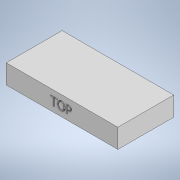
# Autodesk Inventor part: cable_jig_3.5_shim
Saved by Autodesk Inventor 2022 (Build 260153000, 153)
## iProperties
Created: 2022-03-09
Part Number: cable_jig_3.5_shim
Material: Generic
Document SubType Name: Modeling
Designer: kylem
Density: 1 g/cm^3
Appearance: Default
Author: kylem
Autodesk Inventor part; units mm, degrees
ref_plane "YZ Plane" through (0, 0, 0) normal (1, 0, 0) x (0, 1, 0)
ref_plane "XZ Plane" through (0, 0, 0) normal (0, 1, 0) x (-1, 0, 0)
ref_plane "XY Plane" through (0, 0, 0) normal (0, 0, 1) x (1, 0, 0)
sketch "Sketch1" plane through (0, 0, 0) normal (0, 1, 0) x (-1, 0, 0)
  line L0 (0, 0) -> (20, 0)
  line L1 (20, 0) -> (20, -10)
  line L2 (20, -10) -> (0, -10)
  line L3 (0, -10) -> (0, 0)
  dimension "d0" = 20
  dimension "d1" = 10
  constraints: 8 end point, 2 parallel, 1 horizontal, 1 perpendicular
  measures "d0" distance of L1.end L2.end
  measures "d1" distance of L0.end L1.end
extrude "Extrusion1" add sketch "Sketch1" along normal blind 3.45
sketch "Sketch2" plane through (-20, 0, 0) normal (0, 0, 1) x (1, 0, 0)
  line L0 (7.9399, 2.49) -> (16.3941, 2.49) construction
  line L1 (16.3941, 2.49) -> (16.3941, 0.9734) construction
  line L2 (16.3941, 0.9734) -> (7.9399, 0.9734) construction
  line L3 (7.9399, 0.9734) -> (7.9399, 2.49) construction
  line L4 (8.4419, 0.9584) -> (8.4419, 2.2809)
  line L5 (8.4419, 2.2809) -> (7.9386, 2.2809)
  line L6 (7.9386, 2.2809) -> (7.9386, 2.4584)
  line L7 (7.9386, 2.4584) -> (9.1445, 2.4584)
  line L8 (9.1445, 2.4584) -> (9.1445, 2.2809)
  line L9 (9.1445, 2.2809) -> (8.6412, 2.2809)
  line L10 (8.6412, 2.2809) -> (8.6412, 0.9584)
  line L11 (8.6412, 0.9584) -> (8.4419, 0.9584)
  spline S0 degree 2 poles (10.3576, 2.287) (10.4427, 2.1873) (10.5375, 1.8956) (10.5375, 1.7084) knots 0 0 0 1 2 2 2
  spline S1 degree 2 poles (10.5375, 1.7084) (10.5375, 1.526) (10.4451, 1.2307) (10.3576, 1.131) knots 0 0 0 1 2 2 2
  spline S2 degree 2 poles (10.3576, 1.131) (10.2652, 1.0264) (10.0209, 0.9268) (9.8738, 0.9268) knots 0 0 0 1 2 2 2
  spline S3 degree 2 poles (9.8738, 0.9268) (9.7219, 0.9268) (9.4788, 1.0301) (9.39, 1.131) knots 0 0 0 1 2 2 2
  spline S4 degree 2 poles (9.39, 1.131) (9.3037, 1.2307) (9.2113, 1.5236) (9.2113, 1.7084) knots 0 0 0 1 2 2 2
  spline S5 degree 2 poles (9.2113, 1.7084) (9.2113, 1.8968) (9.3049, 2.1837) (9.3912, 2.287) knots 0 0 0 1 2 2 2
  spline S6 degree 2 poles (9.3912, 2.287) (9.4788, 2.3867) (9.7231, 2.49) (9.8738, 2.49) knots 0 0 0 1 2 2 2
  spline S7 degree 2 poles (9.8738, 2.49) (10.027, 2.49) (10.2725, 2.383) (10.3576, 2.287) knots 0 0 0 1 2 2 2
  spline S8 degree 2 poles (10.3296, 1.7084) (10.3296, 1.8567) (10.2652, 2.0864) (10.2069, 2.1618) knots 0 0 0 1 2 2 2
  spline S9 degree 2 poles (10.2069, 2.1618) (10.1473, 2.2396) (9.9796, 2.3174) (9.875, 2.3174) knots 0 0 0 1 2 2 2
  spline S10 degree 2 poles (9.875, 2.3174) (9.7668, 2.3174) (9.604, 2.242) (9.542, 2.1618) knots 0 0 0 1 2 2 2
  spline S11 degree 2 poles (9.542, 2.1618) (9.4824, 2.0852) (9.4192, 1.8542) (9.4192, 1.7084) knots 0 0 0 1 2 2 2
  spline S12 degree 2 poles (9.4192, 1.7084) (9.4192, 1.413) (9.6672, 1.0994) (9.875, 1.0994) knots 0 0 0 1 2 2 2
  spline S13 degree 2 poles (9.875, 1.0994) (10.0829, 1.0994) (10.3296, 1.413) (10.3296, 1.7084) knots 0 0 0 1 2 2 2
  spline S14 degree 2 poles (11.7044, 2.0062) (11.7044, 1.9089) (11.6352, 1.7339) (11.5732, 1.6731) knots 0 0 0 1 2 2 2
  spline S15 degree 2 poles (11.5732, 1.6731) (11.4954, 1.5965) (11.2851, 1.5175) (11.1246, 1.5175) knots 0 0 0 1 2 2 2
  line L12 (11.1246, 1.5175) -> (10.9557, 1.5175)
  line L13 (10.9557, 1.5175) -> (10.9557, 0.9584)
  line L14 (10.9557, 0.9584) -> (10.7563, 0.9584)
  line L15 (10.7563, 0.9584) -> (10.7563, 2.4584)
  line L16 (10.7563, 2.4584) -> (11.1331, 2.4584)
  spline S16 degree 2 poles (11.1331, 2.4584) (11.2668, 2.4584) (11.454, 2.4146) (11.5258, 2.3648) knots 0 0 0 1 2 2 2
  spline S17 degree 2 poles (11.5258, 2.3648) (11.6096, 2.3076) (11.7044, 2.1314) (11.7044, 2.0062) knots 0 0 0 1 2 2 2
  spline S18 degree 2 poles (11.4966, 2.0001) (11.4966, 2.0779) (11.4431, 2.1922) (11.3884, 2.2286) knots 0 0 0 1 2 2 2
  spline S19 degree 2 poles (11.3884, 2.2286) (11.341, 2.2602) (11.2146, 2.2858) (11.121, 2.2858) knots 0 0 0 1 2 2 2
  line L17 (11.121, 2.2858) -> (10.9557, 2.2858)
  line L18 (10.9557, 2.2858) -> (10.9557, 1.6877)
  line L19 (10.9557, 1.6877) -> (11.0918, 1.6877)
  spline S20 degree 2 poles (11.0918, 1.6877) (11.2134, 1.6877) (11.3629, 1.7266) (11.4115, 1.7777) knots 0 0 0 1 2 2 2
  spline S21 degree 2 poles (11.4115, 1.7777) (11.4565, 1.8226) (11.4966, 1.9284) (11.4966, 2.0001) knots 0 0 0 1 2 2 2
  point P0 (20, 0)
  constraints: 2 other
extrude "Extrusion4" cut sketch "Sketch2" against normal blind 0.5
body "Solid1"
